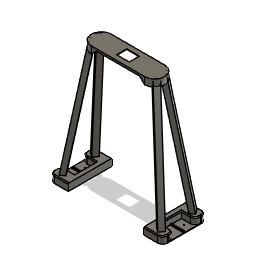
RoboOmnium-merac (Autodesk Fusion 360 design; units mm, degrees)
Autodesk Fusion 360 part; units mm, degrees
sketch "Patky" plane through (0, 0, 0) normal (0, 1, 0) x (1, 0, 0)
  line L0 (148.5, 105) -> (-148.5, 105) construction
  line L1 (-148.5, 105) -> (-148.5, -105) construction
  line L2 (-148.5, -105) -> (148.5, -105) construction
  line L3 (148.5, -105) -> (148.5, 105) construction
  line L4 (148.5, 105) -> (-148.5, -105) construction
  line L5 (-148.5, 105) -> (148.5, -105) construction
  line L6 (184.6496, -69.1462) -> (197.1199, -51.5096)
  line L7 (197.1199, -51.5096) -> (212.4703, -62.3634)
  line L8 (212.4703, -62.3634) -> (200, -80)
  line L9 (200, -80) -> (184.6496, -69.1462)
  line L10 (190.8848, -60.3279) -> (148.5, -30.3588) construction
  line L11 (150, -87.5) -> (225, -87.5)
  line L12 (225, -87.5) -> (225, 87.5)
  line L13 (225, 87.5) -> (150, 87.5)
  line L14 (150, 87.5) -> (150, -87.5)
  line L15 (0, 0) -> (150, 0) construction
  line L16 (170, 42.5) -> (225, 42.5)
  line L17 (225, -42.5) -> (170, -42.5)
  line L18 (170, -42.5) -> (170, 42.5)
  line L19 (197.5, 42.5) -> (197.5, -42.5) construction
  circle A0 centre (197.5, 25) radius 2
  circle A1 centre (197.5, -25) radius 2
  line L20 (170, 2.5) -> (225, 2.5)
  line L21 (170, -2.5) -> (225, -2.5)
  dimension "d1" = 297
  dimension "d2" = 210
  dimension "d3" = 21.6
  dimension "d4" = 18.8
  dimension "d8" = 80
  dimension "d9" = 75
  dimension "d10" = 175
  dimension "d11" = 150
  dimension "d14" = 45
  dimension "d15" = 45
  dimension "d16" = 20
  dimension "d20" = 50
  dimension "d31" = 4
  dimension "d32" = 50
  dimension "d45" = 5
  constraint horizontal L0
  constraint perpendicular L0 L1
  constraint parallel L0 L2
  constraint parallel L1 L3
  constraint coincident L4 L15.start
  constraint coincident L5 L15.start
  constraint coincident L15.start origin
  constraint perpendicular L6 L9
  constraint midpoint L6 L10.start
  constraint perpendicular L6 L10
  constraint parallel L5 L10
  constraint coincident L3 L10.end
  constraint horizontal L11
  constraint vertical L12
  constraint horizontal L13
  constraint vertical L14
  constraint midpoint L14 L15.end
  constraint horizontal L15
  constraint horizontal L16
  constraint horizontal L17
  constraint vertical L18
  constraint coincident L12 L16.end
  constraint coincident L12 L17.start
  constraint midpoint L16 L19.start
  constraint midpoint L17 L19.end
  constraint coincident L19 A0.centre
  constraint symmetric L15 A0 A1
  constraint coincident L18 L20.start
  constraint coincident L12 L20.end
  constraint perpendicular L12 L20
  constraint symmetric L15 L20.start L21.start
  constraint symmetric L15 L20.end L21.end
  measures "d1" distance of L1.end L2.end
  measures "d2" distance of L0.end L1.end
  measures "d3" distance of L7 L9
  measures "d4" distance of L6 L8
  measures "d8" vertical distance of L15.start L8.end
  measures "d9" distance of L11.start L11.end
  measures "d10" distance of L11.start L13.end
  measures "d11" distance of L15.start L14
  measures "d14" distance of L13 L16
  measures "d15" distance of L11 L17
  measures "d16" distance of L14 L18
  measures "d20" distance of L8.end L14
  measures "d31" diameter of A0
  measures "d32" distance of A0.centre A1.centre
  measures "d45" distance of L20 L21
extrude "Extrude1" add sketch "Patky" along normal blind 500 contours L6 L7 L8 L9 makes body 1
move_body "Move1" bodies 1 to x (0.989871, 0.141786, -0.007162) y (-0.141786, 0.984808, -0.100252) z (-0.007162, 0.100252, 0.994936) at (2.3654, -33.1127, 1.6725)
mirror "Mirror1" about plane through (0, 0, 0) normal (0, 0, 1) of bodies 1 makes body 2
mirror "Mirror2" about plane through (0, 0, 0) normal (1, 0, 0) of bodies 1 2 makes body 3 at (-184.4494, 167.3992, 51.3686) makes body 4 at (-184.4494, 167.3992, -51.3686)
ref_plane "WorkPlane1" through (0, 490, 0) normal (0, 1, 0) x (0, 0, 1)
sketch "Preklad" plane through (0, 490, 0) normal (0, 1, 0) x (1, 0, 0)
  line L0 (114.1029, -19.2647) -> (129.6901, -30.2859)
  line L1 (129.6901, -30.2859) -> (142.1605, -12.6493)
  line L2 (142.1605, -12.6493) -> (126.5733, -1.6281)
  line L3 (126.5733, -1.6281) -> (114.1029, -19.2647)
  line L4 (129.6901, 30.2859) -> (114.1029, 19.2647)
  line L5 (114.1029, 19.2647) -> (126.5733, 1.6281)
  line L6 (126.5733, 1.6281) -> (142.1605, 12.6493)
  line L7 (142.1605, 12.6493) -> (129.6901, 30.2859)
  line L8 (-129.6901, -30.2859) -> (-114.1029, -19.2647)
  line L9 (-114.1029, -19.2647) -> (-126.5733, -1.6281)
  line L10 (-126.5733, -1.6281) -> (-142.1605, -12.6493)
  line L11 (-142.1605, -12.6493) -> (-129.6901, -30.2859)
  line L12 (-114.1029, 19.2647) -> (-129.6901, 30.2859)
  line L13 (-129.6901, 30.2859) -> (-142.1605, 12.6493)
  line L14 (-142.1605, 12.6493) -> (-126.5733, 1.6281)
  line L15 (-126.5733, 1.6281) -> (-114.1029, 19.2647)
  line L16 (0, 0) -> (-106.1, 0) construction
  line L17 (0, 0) -> (0, 40) construction
  line L18 (106.1, 40) -> (-106.1, 40)
  line L19 (106.1, -40) -> (-106.1, -40)
  arc A0 (-106.1, 40) -> (-106.1, -40) centre (-106.1, 0) ccw
  arc A1 (106.1, -40) -> (106.1, 40) centre (106.1, 0) ccw
  line L20 (-106.1, 40) -> (-106.1, -40)
  line L21 (106.1, 40) -> (106.1, -40)
  line L22 (25, -20) -> (-25, -20)
  line L23 (-25, -20) -> (-25, 20)
  line L24 (-25, 20) -> (25, 20)
  line L25 (25, 20) -> (25, -20)
  line L26 (25, -20) -> (-25, 20) construction
  line L27 (-25, -20) -> (25, 20) construction
  dimension "d27" = 80
  dimension "d28" = 106.1
  dimension "d29" = 50
  dimension "d30" = 40
  constraint coincident L16.start L17.start
  constraint coincident L16.end A0.centre
  constraint horizontal L16
  constraint perpendicular L16 L17
  constraint symmetric L17 A0 A1
  constraint tangent L18 A0
  constraint tangent L18 A1
  constraint coincident L18 L17.end
  constraint symmetric L16 L18.end L19.end
  constraint symmetric L16 L18.start L19.start
  constraint horizontal L22
  constraint perpendicular L22 L23
  constraint parallel L22 L24
  constraint parallel L23 L25
  constraint coincident L26 L16.start
  constraint coincident L27 L16.start
  measures "d27" diameter of A0
  measures "d28" distance of L16.start L16.end
  measures "d29" distance of L23.end L24.end
  measures "d30" distance of L22.end L23.end
extrude "Extrude2" add sketch "Preklad" along normal blind 8 separate body contours L0 L1 L2 L3 | L4 L5 L6 L7 | L8 L9 L10 L11 | L12 L13 L14 L15 | L18 L19 L20 L21 | A1 L21 | A0 L20 makes body 5
extrude "Extrude3" add sketch "Preklad" against normal blind 20 contours L0 L1 L2 L3 | L4 L5 L6 L7 | L8 L9 L10 L11 | L12 L13 L14 L15 | A1 L21 | A0 L20 bodies 5
chamfer "Chamfer1" distance 20 angle 45 2 edges at (-106.1, 490, 0) (106.1, 490, 0) on bodies 5
chamfer "Chamfer1" distance 6 angle 45 4 edges at (0, 490, 20) (-25, 490, 0) (0, 490, -20) (25, 490, 0) on bodies 5
extrude "Extrude4" add sketch "Patky" against normal blind 2 separate body contours L6 L7 L8 L9 | L11 L12 L13 L14 L16 L17 L18 | L12 L17 L18 L21 | L12 L18 L20 L21 | L12 L16 L18 L20 makes body 6
extrude "Extrude5" add sketch "Patky" along normal blind 26 contours L6 L7 L8 L9 | L11 L12 L13 L14 L16 L17 L18 bodies 6
fillet "Fillet1" radius 20 4 edges at (225, 13, -42.5) (225, 12, -87.5) (225, 13, 42.5) (225, 12, 87.5) on bodies 6
extrude "Extrude6" add sketch "Patky" along normal blind 3.6 contours L12 L18 L20 L21 bodies 6
chamfer "Chamfer2" distance 3.6 angle 45 12 edges at (225, 3.6, 0) (225, 26, -65) (219.1421, 26, -81.6421) (177.5, 26, -87.5) (187.5, 26, -42.5) (219.1421, 26, -48.3579) (170, 26, 0) (225, 26, 65) (219.1421, 26, 48.3579) (187.5, 26, 42.5) (177.5, 26, 87.5) (219.1421, 26, 81.6421) on bodies 6
combine "Combine1" operation cut target body 6 tool bodies 1 2 keep tools
mirror "Mirror3" about plane through (0, 0, 0) normal (1, 0, 0) of bodies 6 makes body 7
combine "Combine2" operation cut target body 5 tool bodies 1 2 3 4 keep tools
named bodies: "Vzpera1", "Vzpera2", "Vzpera3", "Vzpera4", "Preklad", "Patka1", "Patka2"
